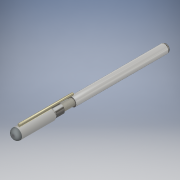
# Autodesk Inventor part: A
Saved by Autodesk Inventor 2017 (Build 210142000, 142)
## iProperties
Part Number: A
Material: 一般
Document SubType Name: Modeling
Designer: user
Density: 1 g/cm^3
Appearance: 鋼 - 拋光
Author: user
Autodesk Inventor part; units mm, degrees
ref_plane "YZ Plane" through (0, 0, 0) normal (1, 0, 0) x (0, 1, 0)
ref_plane "XZ Plane" through (0, 0, 0) normal (0, 1, 0) x (-1, 0, 0)
ref_plane "XY Plane" through (0, 0, 0) normal (0, 0, 1) x (1, 0, 0)
sketch "草圖1" plane through (0, 0, 0) normal (1, 0, 0) x (0, 1, 0)
  line L0 (0, 0) -> (4.5, 0)
  line L1 (4.5, 0) -> (4.5, -100)
  line L2 (4.5, -100) -> (0, -100)
  line L3 (0, -100) -> (0, 0)
  dimension "d3" = 100
  dimension "d4" = 4.5
  constraints: 8 end point, 2 parallel, 1 horizontal, 1 perpendicular
  measures "d3" distance of L2.end L0.start
  measures "d4" distance of L1.end L2.end
revolve "迴轉1" add sketch "草圖1" angle 360 about axis through (0, 0, -100) along (0, 0, 1)
shell "薄殼2" thickness 1 removed faces 1 at (-1.8702, -1.7271, 0)
fillet "圓角3" radius 3 1 edges at (0, -3.5, -99)
fillet "圓角4" radius 3 1 edges at (0, -4.5, -100)
sketch "草圖3" plane through (0, 0, 0) normal (1, 0, 0) x (0, 1, 0)
  line L0 (3.5, 0) -> (3.5, -96) projected
  line L1 (-4.5, 0) -> (4.5, 0) projected
  line L2 (-3.5, 0) -> (-3.5, 12)
  line L3 (-3.5, 12) -> (-4.5, 12)
  line L4 (-4.5, 12) -> (-4.5, 21)
  line L5 (-4.5, 21) -> (-4, 21)
  line L6 (-4, 21) -> (-4, 22)
  line L7 (-4, 22) -> (-4.5, 22)
  line L8 (0, 52) -> (-2, 52)
  arc A0 (-2, 52) -> (-4.5, 22) centre (145.4774, 24.6061) ccw
  line L9 (0, 52) -> (0, 50.2539)
  line L10 (0, 50.2539) -> (0, 0)
  line L11 (-1, 52) -> (-1, 49)
  line L12 (-1, 49) -> (-2, 49)
  line L13 (-2, 49) -> (-2, 0)
  dimension "d20" = 12
  dimension "d21" = 9
  dimension "d22" = 150
  dimension "d23" = 52
  dimension "d24" = 30
  dimension "d26" = 9
  dimension "d27" = 7
  dimension "d28" = 8
  dimension "d29" = 2
  dimension "d30" = 3
  dimension "d31" = 1
  dimension "d32" = 4
  constraints: 24 end point, 6 perpendicular, 3 point on line, 2 point on circle, 2 vertical, 1 centre point, 1 collinear, 1 horizontal, 1 midpoint, 1 parallel
  measures "d20" distance of L2.start L2.end
  measures "d21" distance of L3.end L4.end
  measures "d22" radius of A0
  measures "d23" distance from line of L2.start L8
  measures "d24" distance between parallel lines of L8 L7
  measures "d26" diameter of L4 L10
  measures "d27" diameter of L2 L10
  measures "d28" diameter of L6 L10
  measures "d29" distance of L8.start L8.end
  measures "d30" distance of L11.start L11.end
  measures "d31" distance between parallel lines of L9 L11
  measures "d32" diameter of L13 L10
revolve "迴轉2" add sketch "草圖3" angle 360 about axis through (0, 0, 50.2539) along (0, 0, -1) separate body contours L2 L3 L4 L5 L6 L7 A0 L8 L11 L12 L13 L1
sketch "草圖4" plane through (0, 0, 0) normal (1, 0, 0) x (0, 1, 0)
  line L0 (0, 0) -> (6.3766, 0)
  line L1 (4.5, 22) -> (-4.5, 22) projected
  line L2 (0, 22) -> (5, 22)
  line L3 (5.5, 22.5) -> (5.5, 58)
  line L4 (0, 22) -> (0, 67.5096)
  line L5 (1.5, 62) -> (0, 62)
  line L6 (5, 22) -> (5.5, 22.5)
  arc A0 (5.5, 58) -> (1.5, 62) centre (1.5, 58) ccw
  line L7 (0, 62) -> (0, 22)
  point P0 (5.5, 22)
  point P1 (5.5, 62)
  dimension "d35" = 40
  dimension "d37" = 11
  dimension "d38" = 0.5
  dimension "d39" = 45
  dimension "d40" = 4
  constraints: 14 end point, 5 point on line, 2 horizontal, 2 perpendicular, 2 point on circle, 2 tangent, 2 vertical, 1 centre point, 1 midpoint
  measures "d35" distance of point (5.5, 22) point (5.5, 62)
  measures "d37" diameter of L3 L4
  measures "d38" distance of L2.end point (5.5, 22)
  measures "d39" angle of L2 L6
  measures "d40" radius of A0
revolve "迴轉3" add sketch "草圖4" angle 360 about axis through (0, 0, 62) along (0, 0, -1) separate body
ref_plane "工作平面1" through (0, 0, 56) normal (0, 0, 1) x (1, 0, 0)
sketch "草圖5" plane through (0, 0, 56) normal (0, 0, 1) x (1, 0, 0)
  circle A0 centre (-0.0069, 7) radius 1.25
  point P0 (0, 0)
  dimension "d43" = 2.5
  dimension "d44" = 7
  constraints: 1 centre point
  measures "d43" diameter of A0
  measures "d44" distance of A0.centre point (0, 0)
extrude "擠出2" add sketch "草圖5" against normal blind 57 bodies 3
sketch "草圖7" plane through (-0.0069, 7, 56) normal (0, 0, 1) x (1, 0, 0)
  arc A0 (0.9447, -0.8186) -> (1.2129, -1.6338) centre (1.3226, -1.146) ccw
  arc A1 (-1.2097, -1.6362) -> (-0.9431, -0.8204) centre (-1.3203, -1.1486) ccw
  circle A2 centre (0.0069, -7) radius 5.5 projected
  circle A3 centre (0, 0) radius 1.25 projected
  point P0 (0.0069, -7)
  dimension "d48" = 1
  constraints: 8 point on circle, 4 tangent, 2 centre point, 1 equal radius
  measures "d48" diameter of A1
extrude "擠出3" add sketch "草圖7" against normal up to surface contours A0 A2 A1 A3 round surface about axis through (0, 0, 22.25) along (0, 0, -1) radius 5.25 half angle -45 far side no bodies 3
